Camera Holder Middle (Autodesk Fusion 360 design; units mm, degrees)
Autodesk Fusion 360 part; units mm, degrees
sketch "Sketch1" plane through (0, 0, 0) normal (0, 0, 1) x (1, 0, 0)
  line L0 (-120.55, 25.4) -> (120.65, 25.4)
  line L1 (120.65, 25.4) -> (120.65, -25.4)
  line L2 (120.65, -25.4) -> (-120.55, -25.4)
  line L3 (-120.55, -25.4) -> (-120.55, 25.4)
  dimension "d3" = 241.2
  dimension "d4" = 50.8
  dimension "d5" = 25.4
  dimension "d6" = 120.65
  constraint horizontal L0
  constraint vertical L1
  constraint horizontal L2
  constraint vertical L3
  measures "d3" distance of L1 L3
  measures "d4" distance of L0 L2
  measures "d5" distance of origin L2
  measures "d6" distance of origin L1
extrude "Extrude1" add sketch "Sketch1" along normal blind 2.5
sketch "Sketch2" plane through (0, 0, 2.5) normal (0, 0, 1) x (-1, 0, 0)
  line L0 (120.55, 25.4) -> (-120.65, 25.4)
  line L1 (-120.65, 25.4) -> (-120.65, -25.4)
  line L2 (-120.65, -25.4) -> (120.55, -25.4)
  line L3 (120.55, -25.4) -> (120.55, 25.4)
  line L4 (13.4, -15.4) -> (-13.4, -15.4)
  line L5 (-15.4, -13.4) -> (-15.4, 13.4)
  line L6 (-13.4, 15.4) -> (13.4, 15.4)
  line L7 (15.4, 13.4) -> (15.4, -13.4)
  arc A0 (13.4, -15.4) -> (15.4, -13.4) centre (13.4, -13.4) ccw
  arc A1 (-15.4, -13.4) -> (-13.4, -15.4) centre (-13.4, -13.4) ccw
  arc A2 (-13.4, 15.4) -> (-15.4, 13.4) centre (-13.4, 13.4) ccw
  arc A3 (15.4, 13.4) -> (13.4, 15.4) centre (13.4, 13.4) ccw
  dimension "d7" = 30.8
  dimension "d8" = 30.8
  dimension "d9" = 15.4
  dimension "d10" = 15.4
  dimension "d11" = 2
  constraint horizontal L4
  constraint vertical L5
  constraint horizontal L6
  constraint vertical L7
  constraint tangent L4 A0
  constraint tangent L7 A0
  constraint tangent L4 A1
  constraint tangent L5 A1
  constraint equal A0 A1
  constraint tangent L5 A2
  constraint tangent L6 A2
  constraint equal A0 A2
  constraint tangent L6 A3
  constraint tangent L7 A3
  constraint equal A0 A3
  measures "d7" distance of L5 L7
  measures "d8" distance of L4 L6
  measures "d9" distance of origin L5
  measures "d10" distance of origin L4
  measures "d11" radius of A0
extrude "Extrude2" cut sketch "Sketch2" against normal blind 2.5 contours L4 L5 L6 L7 A0 A1 A2 A3
sketch "Sketch4" plane through (0, 0, 2.5) normal (0, 0, 1) x (-1, 0, 0)
  line L0 (15.4, 13.4) -> (15.4, -13.4)
  arc A0 (13.4, -15.4) -> (15.4, -13.4) centre (13.4, -13.4) ccw
  line L1 (13.4, -15.4) -> (-13.4, -15.4)
  arc A1 (-15.4, -13.4) -> (-13.4, -15.4) centre (-13.4, -13.4) ccw
  line L2 (-15.4, -13.4) -> (-15.4, 13.4)
  arc A2 (-13.4, 15.4) -> (-15.4, 13.4) centre (-13.4, 13.4) ccw
  line L3 (-13.4, 15.4) -> (13.4, 15.4)
  arc A3 (15.4, 13.4) -> (13.4, 15.4) centre (13.4, 13.4) ccw
  line L4 (120.55, 25.4) -> (-120.65, 25.4)
  line L5 (-120.65, 25.4) -> (-120.65, -25.4)
  line L6 (-120.65, -25.4) -> (120.55, -25.4)
  line L7 (120.55, -25.4) -> (120.55, 25.4)
  line L8 (18, -20) -> (-18, -20)
  line L9 (-20, -18) -> (-20, 18)
  line L10 (-18, 20) -> (18, 20)
  line L11 (20, 18) -> (20, -18)
  arc A4 (18, -20) -> (20, -18) centre (18, -18) ccw
  arc A5 (-20, -18) -> (-18, -20) centre (-18, -18) ccw
  arc A6 (-18, 20) -> (-20, 18) centre (-18, 18) ccw
  arc A7 (20, 18) -> (18, 20) centre (18, 18) ccw
  dimension "d18" = 40
  dimension "d19" = 40
  dimension "d20" = 20
  dimension "d21" = 20
  dimension "d22" = 2
  constraint horizontal L8
  constraint vertical L9
  constraint horizontal L10
  constraint vertical L11
  constraint tangent L8 A4
  constraint tangent L11 A4
  constraint tangent L8 A5
  constraint tangent L9 A5
  constraint equal A4 A5
  constraint tangent L9 A6
  constraint tangent L10 A6
  constraint equal A4 A6
  constraint tangent L10 A7
  constraint tangent L11 A7
  constraint equal A4 A7
  measures "d18" distance of L9 L11
  measures "d19" distance of L8 L10
  measures "d20" distance of origin L9
  measures "d21" distance of origin L8
  measures "d22" radius of A4
extrude "Extrude3" add sketch "Sketch4" along normal blind 2.5 contours L8 L9 L10 L11 A4 A5 A6 A7
sketch "Sketch6" plane through (0, 0, 5) normal (0, 0, 1) x (-1, 0, 0)
  arc A0 (13.4, -15.4) -> (15.4, -13.4) centre (13.4, -13.4) ccw
  line L0 (13.4, -15.4) -> (-13.4, -15.4)
  arc A1 (-15.4, -13.4) -> (-13.4, -15.4) centre (-13.4, -13.4) ccw
  line L1 (-15.4, -13.4) -> (-15.4, 13.4)
  arc A2 (-13.4, 15.4) -> (-15.4, 13.4) centre (-13.4, 13.4) ccw
  line L2 (-13.4, 15.4) -> (13.4, 15.4)
  arc A3 (15.4, 13.4) -> (13.4, 15.4) centre (13.4, 13.4) ccw
  line L3 (15.4, 13.4) -> (15.4, -13.4)
  arc A4 (18, -20) -> (20, -18) centre (18, -18) ccw
  line L4 (20, -18) -> (20, 18)
  arc A5 (20, 18) -> (18, 20) centre (18, 18) ccw
  line L5 (18, 20) -> (-18, 20)
  arc A6 (-18, 20) -> (-20, 18) centre (-18, 18) ccw
  line L6 (-20, 18) -> (-20, -18)
  arc A7 (-20, -18) -> (-18, -20) centre (-18, -18) ccw
  line L7 (-18, -20) -> (18, -20)
  point P0 (17, -17)
  point P1 (-17, -17)
  point P2 (-17, 17)
  point P3 (17, 17)
  dimension "d29" = 34
  dimension "d30" = 34
  dimension "d31" = 17
  dimension "d32" = 17
  constraint horizontal P0 P1
  constraint vertical P1 P2
  constraint horizontal P2 P3
  constraint vertical P0 P3
  measures "d29" horizontal distance of P0 P1
  measures "d30" vertical distance of P1 P2
  measures "d31" horizontal distance of origin P1
  measures "d32" vertical distance of origin P1
hole "Hole1" at (-17, 17, 5) at (17, 17, 5) at (17, -17, 5) at (-17, -17, 5) direction (0, 0, -1) diameter 2.54 depth 5 tip angle 118
chamfer "Chamfer1" distance 2.5 distance2 2.5 8 edges at (0, -20, 2.5) (-19.4142, -19.4142, 2.5) (-20, 0, 2.5) (-19.4142, 19.4142, 2.5) (0, 20, 2.5) (19.4142, 19.4142, 2.5) (20, 0, 2.5) (19.4142, -19.4142, 2.5) measured on face at (87.1, -6, 2.5) measured on face at (87.1, -6, 2.5) measured on face at (87.1, -6, 2.5) measured on face at (87.1, -6, 2.5) measured on face at (87.1, -6, 2.5) measured on face at (87.1, -6, 2.5) measured on face at (87.1, -6, 2.5) measured on face at (87.1, -6, 2.5)
fillet "Fillet1" radius 2.5 8 edges at (22.5, 0, 2.5) (21.182, 21.182, 2.5) (0, 22.5, 2.5) (-21.182, 21.182, 2.5) (-22.5, 0, 2.5) (-21.182, -21.182, 2.5) (0, -22.5, 2.5) (21.182, -21.182, 2.5)
sketch "Sketch7" plane through (0, 0, 0) normal (0, 0, -1) x (1, 0, 0)
  circle A0 centre (17, 17) radius 1.27
  circle A1 centre (-17, -17) radius 1.27
  circle A2 centre (17, -17) radius 1.27
  circle A3 centre (-17, 17) radius 1.27
  line L0 (-15.4, -13.4) -> (-15.4, 13.4)
  arc A4 (-13.4, 15.4) -> (-15.4, 13.4) centre (-13.4, 13.4) ccw
  line L1 (-13.4, 15.4) -> (13.4, 15.4)
  arc A5 (15.4, 13.4) -> (13.4, 15.4) centre (13.4, 13.4) ccw
  line L2 (15.4, 13.4) -> (15.4, -13.4)
  arc A6 (13.4, -15.4) -> (15.4, -13.4) centre (13.4, -13.4) ccw
  line L3 (13.4, -15.4) -> (-13.4, -15.4)
  arc A7 (-15.4, -13.4) -> (-13.4, -15.4) centre (-13.4, -13.4) ccw
  line L4 (120.65, 25.4) -> (-120.55, 25.4)
  line L5 (-120.55, 25.4) -> (-120.55, -25.4)
  line L6 (-120.55, -25.4) -> (120.65, -25.4)
  line L7 (120.65, -25.4) -> (120.65, 25.4)
  point P0 (-112.9, 15)
  point P1 (-112.9, -15)
  point P2 (113, 15)
  point P3 (113, -15)
  dimension "d40" = 30
  dimension "d41" = 7.65
  dimension "d42" = 7.65
  dimension "d48" = 10.4
  constraint horizontal P0 P2
  constraint vertical P2 P3
  constraint horizontal P1 P3
  constraint vertical P0 P1
  measures "d40" distance of P0 P1
  measures "d41" distance of L5 P0
  measures "d42" distance of L7 P2
  measures "d48" distance of L4 P0
hole "Hole2" at (-112.9, -15, 0) at (-112.9, 15, 0) at (113, -15, 0) at (113, 15, 0) direction (0, 0, 1) diameter 4.5 depth 5 tip angle 180 countersink diameter 9.4 countersink angle 90
extrude "Extrude5" add 1 faces at (-17.0425, 4.4667, 5) along direction (0, 0, 1) blind 10
equation "d3 = 9.5 in - 0.1 mm"
equation "d6 = ( 9.5 / 2 ) * 1 in"
equation "d41 = ( ( 15.4 / 2 ) * 1 mm ) - 0.05 * 1 mm"
equation "d42 = ( ( 15.4 / 2 ) * 1 mm ) - 0.05 * 1 mm"
equation "d48 = ( 2 in - 30 mm ) / 2"
